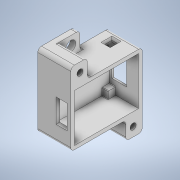
# Autodesk Inventor part: gehaeuse_wemos
Saved by Autodesk Inventor 2020 (Build 240168000, 168)
## iProperties
Created: 2020-05-23
Part Number: gehaeuse_wemos
Material: Generisch
Document SubType Name: Modeling
Designer: chris
Density: 1 g/cm^3
Appearance: Vorgabe
Author: chris
Autodesk Inventor part; units mm, degrees
ref_plane "YZ Plane" through (0, 0, 0) normal (1, 0, 0) x (0, 1, 0)
ref_plane "XZ Plane" through (0, 0, 0) normal (0, 1, 0) x (-1, 0, 0)
ref_plane "XY Plane" through (0, 0, 0) normal (0, 0, 1) x (1, 0, 0)
sketch "Skizze1" plane through (0, 0, 0) normal (1, 0, 0) x (0, 1, 0)
  line L0 (0, 0) -> (30, 0)
  line L1 (30, 0) -> (30, -39)
  line L2 (30, -39) -> (0, -39)
  line L3 (0, -39) -> (0, 0)
  dimension "d0" = 39
  dimension "d1" = 30
  constraints: 8 end point, 2 parallel, 1 horizontal, 1 perpendicular
  measures "d0" distance of L2.end L0.start
  measures "d1" distance of L0.start L0.end
extrude "Extrusion1" add sketch "Skizze1" along normal blind 18
shell "Wandung1" thickness 2 removed faces 1 at (18, 10, -13)
sketch "Skizze2" plane through (2, 2, -37) normal (1, 0, 0) x (0, 0, -1)
  line L0 (-35, 26) -> (-35, 0) projected
  line L1 (-35, 26) -> (-31, 26)
  line L2 (-31, 26) -> (-31, 22)
  line L3 (-31, 22) -> (-35, 22)
  line L4 (-35, 22) -> (-35, 26)
  line L5 (0, 26) -> (0, 0) projected
  line L6 (0, 26) -> (-4, 26)
  line L7 (-4, 26) -> (-4, 22)
  line L8 (-4, 22) -> (0, 22)
  line L9 (0, 22) -> (0, 26)
  line L10 (0, 0) -> (-4, 0)
  line L11 (-4, 0) -> (-4, 4)
  line L12 (-4, 4) -> (0, 4)
  line L13 (0, 4) -> (0, 0)
  line L14 (-35, 0) -> (0, 0) projected
  line L15 (-35, 0) -> (-31, 0)
  line L16 (-31, 0) -> (-31, 4)
  line L17 (-31, 4) -> (-35, 4)
  line L18 (-35, 4) -> (-35, 0)
  point P0 (-37, -2)
  point P1 (-35, 4)
  point P2 (-31, 0)
  point P3 (0, 4)
  point P4 (0, 22)
  dimension "d5" = 4
  dimension "d6" = 4
  dimension "d7" = 4
  dimension "d8" = 4
  constraints: 32 end point, 8 parallel, 4 horizontal, 4 perpendicular, 4 point on line
  measures "d5" distance of L2.end L3.end
  measures "d6" distance between parallel lines of L1 L3
  measures "d7" distance between parallel lines of L5 L7
  measures "d8" distance between parallel lines of L10 L12
extrude "Extrusion2" add sketch "Skizze2" along normal blind 3.5
fillet "Rundung1" radius 0.3 12 edges at (3.75, 24, -6) (3.75, 24, -2) (3.75, 28, -6) (3.75, 28, -33) (3.75, 24, -33) (3.75, 24, -37) (3.75, 6, -37) (3.75, 6, -33) (3.75, 2, -33) (3.75, 6, -2) (3.75, 6, -6) (3.75, 2, -6)
sketch "Skizze3" plane through (0, 0, -39) normal (0, 0, -1) x (-1, 0, 0)
  line L0 (-10.5, 20) -> (-6.5, 20)
  line L1 (-6.5, 20) -> (-6.5, 11)
  line L2 (-6.5, 11) -> (-10.5, 11)
  line L3 (-10.5, 11) -> (-10.5, 20)
  line L4 (0, 30) -> (-18, 30) projected
  line L5 (0, 0) -> (-18, 0) projected
  line L6 (0, 0) -> (0, 30) projected
  dimension "d12" = 9
  dimension "d13" = 4
  dimension "d15" = 11
  dimension "d16" = 6.5
  constraints: 8 end point, 2 parallel, 1 horizontal, 1 perpendicular
  measures "d12" distance between parallel lines of L2 L0
  measures "d13" distance between parallel lines of L1 L3
  measures "d15" distance between parallel lines of L5 L2
  measures "d16" distance between parallel lines of L6 L1
extrude "Extrusion3" cut sketch "Skizze3" against normal blind 3.5
sketch "Skizze4" plane through (0, 0, -39) normal (0, 0, -1) x (-1, 0, 0)
  line L0 (-11.5, 9) -> (-3.5, 9)
  line L1 (-3.5, 9) -> (-3.5, 22)
  line L2 (-3.5, 22) -> (-11.5, 22)
  line L3 (-11.5, 22) -> (-11.5, 9)
  line L4 (-10.5, 11) -> (-10.5, 20) projected
  line L5 (-6.5, 11) -> (-10.5, 11) projected
  point P0 (0, 0)
  dimension "d19" = 1
  dimension "d20" = 8
  dimension "d21" = 13
  dimension "d22" = 2
  constraints: 8 end point, 2 parallel, 1 horizontal, 1 perpendicular
  measures "d19" distance between parallel lines of L3 L4
  measures "d20" distance between parallel lines of L1 L3
  measures "d21" distance between parallel lines of L2 L0
  measures "d22" distance between parallel lines of L0 L5
extrude "Extrusion4" cut sketch "Skizze4" against normal blind 2
sketch "Skizze5" plane through (0, 0, 0) normal (0, 0, 1) x (1, 0, 0)
  line L0 (16, 22) -> (10, 22)
  line L1 (10, 22) -> (10, 9)
  line L2 (10, 9) -> (16, 9)
  line L3 (16, 9) -> (16, 22)
  line L4 (18, 30) -> (18, 0) projected
  line L5 (0, 30) -> (18, 30) projected
  point P0 (0, 0)
  dimension "d25" = 13
  dimension "d26" = 6
  dimension "d27" = 2
  dimension "d28" = 8
  constraints: 8 end point, 2 parallel, 1 horizontal, 1 perpendicular
  measures "d25" distance between parallel lines of L0 L2
  measures "d26" distance between parallel lines of L1 L3
  measures "d27" distance between parallel lines of L4 L3
  measures "d28" distance between parallel lines of L5 L0
extrude "Extrusion5" cut sketch "Skizze5" against normal blind 2
sketch "Skizze6" plane through (0, 30, 0) normal (0, 1, 0) x (1, 0, 0)
  line L0 (8.5, 31) -> (5.5, 31)
  line L1 (5.5, 31) -> (5.5, 35)
  line L2 (5.5, 35) -> (8.5, 35)
  line L3 (8.5, 35) -> (8.5, 31)
  line L4 (0, 39) -> (18, 39) projected
  line L5 (0, 39) -> (0, 0) projected
  dimension "d31" = 3
  dimension "d32" = 4
  dimension "d33" = 4
  dimension "d34" = 5.5
  constraints: 8 end point, 2 parallel, 1 horizontal, 1 perpendicular
  measures "d31" distance between parallel lines of L1 L3
  measures "d32" distance between parallel lines of L0 L2
  measures "d33" distance between parallel lines of L4 L2
  measures "d34" distance between parallel lines of L5 L1
extrude "Extrusion6" cut sketch "Skizze6" against normal blind 2
chamfer "Fase1" distance 1 angle 45 4 edges at (5.5, 30, -33) (7, 30, -31) (7, 30, -35) (8.5, 30, -33)
chamfer "Fase2" distance 1 angle 45 4 edges at (3.5, 15.5, -39) (7.5, 9, -39) (11.5, 15.5, -39) (7.5, 22, -39)
sketch "Skizze7" plane through (0, 0, 0) normal (-1, 0, 0) x (0, 0, 1)
  line L0 (0, 0) -> (-39, 0) projected
  line L1 (-39, 30) -> (0, 30) projected
  line L2 (0, 30) -> (-20, 30)
  line L3 (-20, 30) -> (-20, 40)
  line L4 (-20, 40) -> (0, 40)
  line L5 (0, 40) -> (0, 30)
  line L6 (-39, 0) -> (-19, 0)
  line L7 (-19, 0) -> (-19, -10)
  line L8 (-19, -10) -> (-39, -10)
  line L9 (-39, -10) -> (-39, 0)
  dimension "d43" = 10
  dimension "d44" = 20
  dimension "d45" = 20
  dimension "d46" = 10
  constraints: 16 end point, 4 parallel, 2 horizontal, 2 perpendicular
  measures "d43" distance between parallel lines of L0 L8
  measures "d44" distance between parallel lines of L9 L7
  measures "d45" distance between parallel lines of L5 L3
  measures "d46" distance between parallel lines of L1 L4
extrude "Extrusion7" add sketch "Skizze7" against normal blind 3
sketch "Skizze8" plane through (0, 0, 0) normal (-1, 0, 0) x (0, 0, 1)
  line L0 (-2.1, 36.6743) -> (-2.1, 33.3257)
  line L1 (-2.1, 33.3257) -> (-5, 31.6514)
  line L2 (-5, 31.6514) -> (-7.9, 33.3257)
  line L3 (-7.9, 33.3257) -> (-7.9, 36.6743)
  line L4 (-7.9, 36.6743) -> (-5, 38.3486)
  line L5 (-5, 38.3486) -> (-2.1, 36.6743)
  line L6 (-31.1, -6.6743) -> (-34, -8.3486)
  line L7 (-34, -8.3486) -> (-36.9, -6.6743)
  line L8 (-36.9, -6.6743) -> (-36.9, -3.3257)
  line L9 (-36.9, -3.3257) -> (-34, -1.6514)
  line L10 (-34, -1.6514) -> (-31.1, -3.3257)
  line L11 (-31.1, -3.3257) -> (-31.1, -6.6743)
  line L12 (0, 0) -> (0, 40) projected
  line L13 (0, 40) -> (-20, 40) projected
  line L14 (-39, -10) -> (-39, 30) projected
  line L15 (-39, -10) -> (-19, -10) projected
  circle A0 centre (-24, -5) radius 2.75
  circle A1 centre (-15, 35) radius 2.75
  line L16 (-19, -10) -> (-19, 0) projected
  line L17 (-20, 40) -> (-20, 30) projected
  point P0 (-5, 35)
  point P1 (-34, -5)
  dimension "d49" = 5.8
  dimension "d50" = 5
  dimension "d51" = 5
  dimension "d52" = 5
  dimension "d53" = 5.8
  dimension "d54" = 5
  dimension "d57" = 5.5
  dimension "d58" = 5
  dimension "d59" = 5
  dimension "d60" = 5
  dimension "d61" = 5
  constraints: 24 end point, 2 centre point, 2 vertical, 1 equal radius, 26 other
  measures "d49" distance between parallel lines of L1 L4
  measures "d50" distance from line of L12 point (-5, 35)
  measures "d51" distance from line of L13 point (-5, 35)
  measures "d52" distance from line of L14 point (-34, -5)
  measures "d53" distance between parallel lines of L9 L6
  measures "d54" distance from line of L15 point (-34, -5)
  measures "d57" diameter of A0
  measures "d58" distance from line of L16 A0.centre
  measures "d59" distance from line of L15 A0.centre
  measures "d60" distance from line of L17 A1.centre
  measures "d61" distance from line of L13 A1.centre
extrude "Extrusion8" cut sketch "Skizze8" against normal blind 3
sketch "Skizze9" plane through (3, 0, 0) normal (1, 0, 0) x (0, 0, -1)
  line L0 (19, 0) -> (39, 0) projected
  line L1 (39, -10) -> (30, -10)
  line L2 (30, -10) -> (30, 0)
  line L3 (30, 0) -> (39, 0)
  line L4 (39, 0) -> (39, -10)
  line L5 (19, -10) -> (39, -10) projected
  line L6 (0, 0) -> (0, 40) projected
  line L7 (39, 30) -> (0, 30) projected
  line L8 (0, 40) -> (9, 40)
  line L9 (9, 40) -> (9, 30)
  line L10 (9, 30) -> (0, 30)
  line L11 (0, 30) -> (0, 40)
  line L12 (39, -10) -> (39, 0) projected
  dimension "d62" = 9
  dimension "d63" = 9
  constraints: 16 end point, 4 parallel, 2 collinear, 2 horizontal, 2 perpendicular, 2 point on line
  measures "d62" distance between parallel lines of L6 L9
  measures "d63" distance between parallel lines of L4 L2
extrude "Extrusion9" add sketch "Skizze9" along normal blind 15
sketch "Skizze10" plane through (18, 0, 0) normal (1, 0, 0) x (0, 0, -1)
  circle A0 centre (34, -5) radius 1.65
  line L0 (39, -10) -> (39, 30) projected
  line L1 (30, -10) -> (39, -10) projected
  circle A1 centre (5, 35) radius 1.65
  line L2 (0, 40) -> (0, 0) projected
  line L3 (9, 40) -> (0, 40) projected
  dimension "d66" = 5
  dimension "d67" = 3.3
  dimension "d68" = 5
  dimension "d69" = 5
  dimension "d70" = 5
  dimension "d71" = 3.3
  constraints: 2 centre point
  measures "d66" distance from line of L0 A0.centre
  measures "d67" diameter of A0
  measures "d68" distance from line of L1 A0.centre
  measures "d69" distance from line of L2 A1.centre
  measures "d70" distance from line of L3 A1.centre
  measures "d71" diameter of A1
extrude "Extrusion10" cut sketch "Skizze10" against normal blind 19
fillet "Rundung2" radius 2 10 edges at (9, 0, 0) (9, 30, -39) (10.5, -10, -30) (1.5, -10, -19) (1.5, 0, -19) (1.5, 30, -20) (1.5, 40, -20) (10.5, 40, -9) (10.5, 0, -30) (10.5, 30, -9)
